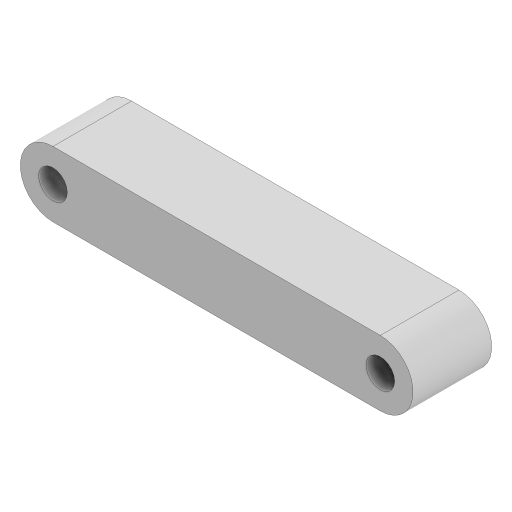
# Autodesk Inventor part: Neck Servo Arm
Saved by Autodesk Inventor 2024 (Build 280153000, 153)
## iProperties
Created: 2025-04-26
Part Number: Neck Servo Arm
Material: Generic
Document SubType Name: Modeling
Designer: Binara
Density: 1 g/cm^3
Appearance: Default
Author: Binara
## iProperties of the stored document Neck Servo Arm_3DPrint.ipt
Created: 2025-04-26
Part Number: Neck Servo Arm_3DPrint
Material: Generic
Document SubType Name: Modeling
Designer: Binara
Density: 1 g/cm^3
Appearance: Default
Author: Binara
Autodesk Inventor part; units mm, degrees
ref_plane "YZ Plane" through (0, 0, 0) normal (1, 0, 0) x (0, 1, 0)
ref_plane "XZ Plane" through (0, 0, 0) normal (0, 1, 0) x (-1, 0, 0)
ref_plane "XY Plane" through (0, 0, 0) normal (0, 0, 1) x (1, 0, 0)
sketch "Sketch1" plane through (0, 0, 0) normal (0, 0, 1) x (1, 0, 0)
  line L0 (-20, 0) -> (20, 0) construction
  line L1 (-20, -4) -> (20, -4)
  line L2 (20, 4) -> (-20, 4)
  arc A0 (-20, 4) -> (-20, -4) centre (-20, 0) ccw
  arc A1 (20, -4) -> (20, 4) centre (20, 0) ccw
  circle A2 centre (20, 0) radius 1.75
  circle A3 centre (-20, 0) radius 1.75
  point P0 (0, 0)
  dimension "d0" = 20
  dimension "d1" = 8
  dimension "d2" = 3.5
  dimension "d3" = 3.5
  constraints: 8 end point, 4 centre point, 4 point on circle, 4 tangent, 2 coincident, 1 horizontal, 1 midpoint, 1 parallel
  measures "d0" distance of point (0, 0) L0.end
  measures "d1" diameter of A1
  measures "d2" diameter of A2
  measures "d3" diameter of A3
extrude "Extrusion1" add sketch "Sketch1" along normal blind 9.607
body "Solid1"
